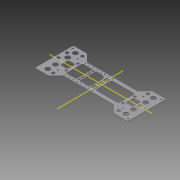
# Autodesk Inventor part: piastraX
Saved by Autodesk Inventor 2014 SP1 (Build 180222100, 222)
## iProperties
Created: 2015-04-08
Part Number: piastraX
Material: Generic
Document SubType Name: Modeling
Designer: Giorgio Nuzzo
Density: 1 g/cm^3
Appearance: Default
Author: Giorgio Nuzzo
Autodesk Inventor part; units mm, degrees
(part 1 of 6)
ref_plane "YZ Plane" through (0, 0, 0) normal (1, 0, 0) x (0, 1, 0)
ref_plane "XZ Plane" through (0, 0, 0) normal (0, 1, 0) x (-1, 0, 0)
ref_plane "XY Plane" through (0, 0, 0) normal (0, 0, 1) x (1, 0, 0)
sketch "Sketch1" plane through (0, 0, 0) normal (0, 0, 1) x (1, 0, 0)
  line L0 (224.6643, 218.6959) -> (272.1277, 218.6959)
  spline S0 degree 3 poles (272.1277, 218.6959) (273.7845, 218.6959) (275.1277, 217.3526) (275.1277, 215.6959) knots 1 1 1 1 2 2 2 2
  line L1 (272.1277, 218.6959) -> (273.7845, 218.6959) construction
  line L2 (273.7845, 218.6959) -> (275.1277, 217.3526) construction
  line L3 (275.1277, 217.3526) -> (275.1277, 215.6959) construction
  line L4 (275.1277, 215.6959) -> (275.1277, 81.696)
  spline S1 degree 3 poles (275.1277, 81.696) (275.1277, 80.0389) (273.7845, 78.696) (272.1277, 78.696) knots 3 3 3 3 4 4 4 4
  line L5 (275.1277, 81.696) -> (275.1277, 80.0389) construction
  line L6 (275.1277, 80.0389) -> (273.7845, 78.696) construction
  line L7 (273.7845, 78.696) -> (272.1277, 78.696) construction
  line L8 (272.1277, 78.696) -> (224.6664, 78.696)
  line L9 (224.6664, 78.696) -> (197.1053, 106.2571)
  line L10 (197.1053, 106.2571) -> (12.6874, 106.2571)
  line L11 (12.6874, 106.2571) -> (-14.8739, 78.696)
  line L12 (-14.8739, 78.696) -> (-61.8722, 78.696)
  spline S2 degree 3 poles (-61.8722, 78.696) (-63.5291, 78.696) (-64.8722, 80.0389) (-64.8722, 81.696) (-64.8722, 81.696) (-64.8722, 215.6959) (-64.8722, 215.6959) (-64.8722, 217.3526) (-63.5291, 218.6959) (-61.8722, 218.6959) knots 9 9 9 9 10 10 10 11 11 11 12 12 12 12
  line L13 (-61.8722, 78.696) -> (-63.5291, 78.696) construction
  line L14 (-63.5291, 78.696) -> (-64.8722, 80.0389) construction
  line L15 (-64.8722, 80.0389) -> (-64.8722, 81.696) construction
  line L16 (-64.8722, 81.696) -> (-64.8722, 81.696) construction
  line L17 (-64.8722, 81.696) -> (-64.8722, 215.6959) construction
  line L18 (-64.8722, 215.6959) -> (-64.8722, 215.6959) construction
  line L19 (-64.8722, 215.6959) -> (-64.8722, 217.3526) construction
  line L20 (-64.8722, 217.3526) -> (-63.5291, 218.6959) construction
  line L21 (-63.5291, 218.6959) -> (-61.8722, 218.6959) construction
  line L22 (-61.8722, 218.6959) -> (-14.8718, 218.6959)
  line L23 (-14.8718, 218.6959) -> (12.6282, 191.1959)
  line L24 (12.6282, 191.1959) -> (197.1645, 191.1959)
  line L25 (197.1645, 191.1959) -> (224.6643, 218.6959)
  line L26 (-42.132, 147.4797) -> (-42.132, 158.9796)
  line L27 (-42.132, 158.9796) -> (-37.8194, 150.7141)
  line L28 (-37.8194, 150.7141) -> (-33.507, 158.9796)
  line L29 (-33.507, 158.9796) -> (-33.507, 147.4797)
  line L30 (-60.4222, 87.8958) -> (-60.4065, 88.2075)
  line L31 (-60.4065, 88.2075) -> (-60.3603, 88.5104)
  line L32 (-60.3603, 88.5104) -> (-60.285, 88.8028)
  line L33 (-60.285, 88.8028) -> (-60.1825, 89.0829)
  line L34 (-60.1825, 89.0829) -> (-60.054, 89.3496)
  line L35 (-60.054, 89.3496) -> (-59.9013, 89.6011)
  line L36 (-59.9013, 89.6011) -> (-59.7257, 89.836)
  line L37 (-59.7257, 89.836) -> (-59.5288, 90.0524)
  line L38 (-59.5288, 90.0524) -> (-59.3123, 90.2494)
  line L39 (-59.3123, 90.2494) -> (-59.0775, 90.4248)
  line L40 (-59.0775, 90.4248) -> (-58.826, 90.5778)
  line L41 (-58.826, 90.5778) -> (-58.5594, 90.7063)
  line L42 (-58.5594, 90.7063) -> (-58.2791, 90.8086)
  line L43 (-58.2791, 90.8086) -> (-57.987, 90.884)
  line L44 (-57.987, 90.884) -> (-57.684, 90.9302)
  line L45 (-57.684, 90.9302) -> (-57.3722, 90.9457)
  line L46 (-57.3722, 90.9457) -> (-57.0604, 90.9302)
  line L47 (-57.0604, 90.9302) -> (-56.7576, 90.884)
  line L48 (-56.7576, 90.884) -> (-56.4653, 90.8086)
  line L49 (-56.4653, 90.8086) -> (-56.185, 90.7063)
  line L50 (-56.185, 90.7063) -> (-55.9184, 90.5778)
  line L51 (-55.9184, 90.5778) -> (-55.6669, 90.4248)
  line L52 (-55.6669, 90.4248) -> (-55.4321, 90.2494)
  line L53 (-55.4321, 90.2494) -> (-55.2156, 90.0524)
  line L54 (-55.2156, 90.0524) -> (-55.0187, 89.836)
  line L55 (-55.0187, 89.836) -> (-54.8432, 89.6011)
  line L56 (-54.8432, 89.6011) -> (-54.6904, 89.3496)
  line L57 (-54.6904, 89.3496) -> (-54.5619, 89.0829)
  line L58 (-54.5619, 89.0829) -> (-54.4594, 88.8028)
  line L59 (-54.4594, 88.8028) -> (-54.3841, 88.5104)
  line L60 (-54.3841, 88.5104) -> (-54.3379, 88.2075)
  line L61 (-54.3379, 88.2075) -> (-54.3223, 87.8958)
  line L62 (-54.3223, 87.8958) -> (-54.3379, 87.584)
  line L63 (-54.3379, 87.584) -> (-54.3841, 87.2811)
  line L64 (-54.3841, 87.2811) -> (-54.4594, 86.989)
  line L65 (-54.4594, 86.989) -> (-54.5619, 86.7086)
  line L66 (-54.5619, 86.7086) -> (-54.6904, 86.4419)
  line L67 (-54.6904, 86.4419) -> (-54.8432, 86.1904)
  line L68 (-54.8432, 86.1904) -> (-55.0187, 85.9558)
  line L69 (-55.0187, 85.9558) -> (-55.2156, 85.7391)
  line L70 (-55.2156, 85.7391) -> (-55.4321, 85.5424)
  line L71 (-55.4321, 85.5424) -> (-55.6669, 85.3667)
  line L72 (-55.6669, 85.3667) -> (-55.9184, 85.2141)
  line L73 (-55.9184, 85.2141) -> (-56.185, 85.0856)
  line L74 (-56.185, 85.0856) -> (-56.4653, 84.9829)
  line L75 (-56.4653, 84.9829) -> (-56.7576, 84.9078)
  line L76 (-56.7576, 84.9078) -> (-57.0604, 84.8617)
  line L77 (-57.0604, 84.8617) -> (-57.3722, 84.8458)
  line L78 (-57.3722, 84.8458) -> (-57.684, 84.8617)
  line L79 (-57.684, 84.8617) -> (-57.987, 84.9078)
  line L80 (-57.987, 84.9078) -> (-58.2791, 84.9829)
  line L81 (-58.2791, 84.9829) -> (-58.5594, 85.0856)
  line L82 (-58.5594, 85.0856) -> (-58.826, 85.2141)
  line L83 (-58.826, 85.2141) -> (-59.0775, 85.3667)
  line L84 (-59.0775, 85.3667) -> (-59.3123, 85.5424)
  line L85 (-59.3123, 85.5424) -> (-59.5288, 85.7391)
  line L86 (-59.5288, 85.7391) -> (-59.7257, 85.9558)
  line L87 (-59.7257, 85.9558) -> (-59.9013, 86.1904)
  line L88 (-59.9013, 86.1904) -> (-60.054, 86.4419)
  line L89 (-60.054, 86.4419) -> (-60.1825, 86.7086)
  line L90 (-60.1825, 86.7086) -> (-60.285, 86.989)
  line L91 (-60.285, 86.989) -> (-60.3603, 87.2811)
  line L92 (-60.3603, 87.2811) -> (-60.4065, 87.584)
  line L93 (-60.4065, 87.584) -> (-60.4222, 87.8958)
  line L94 (-59.4222, 96.1919) -> (-59.4117, 96.4014)
  line L95 (-59.4117, 96.4014) -> (-59.3805, 96.605)
  line L96 (-59.3805, 96.605) -> (-59.3301, 96.8013)
  line L97 (-59.3301, 96.8013) -> (-59.2612, 96.9898)
  line L98 (-59.2612, 96.9898) -> (-59.1749, 97.1689)
  line L99 (-59.1749, 97.1689) -> (-59.0722, 97.3381)
  line L100 (-59.0722, 97.3381) -> (-58.954, 97.4959)
  line L101 (-58.954, 97.4959) -> (-58.8217, 97.6412)
  line L102 (-58.8217, 97.6412) -> (-58.6762, 97.7739)
  line L103 (-58.6762, 97.7739) -> (-58.5184, 97.8917)
  line L104 (-58.5184, 97.8917) -> (-58.3494, 97.9944)
  line L105 (-58.3494, 97.9944) -> (-58.1701, 98.0808)
  line L106 (-58.1701, 98.0808) -> (-57.9818, 98.1497)
  line L107 (-57.9818, 98.1497) -> (-57.7854, 98.2)
  line L108 (-57.7854, 98.2) -> (-57.5818, 98.2314)
  line L109 (-57.5818, 98.2314) -> (-57.3722, 98.2417)
  line L110 (-57.3722, 98.2417) -> (-57.1626, 98.2314)
  line L111 (-57.1626, 98.2314) -> (-56.9591, 98.2)
  line L112 (-56.9591, 98.2) -> (-56.7626, 98.1497)
  line L113 (-56.7626, 98.1497) -> (-56.5743, 98.0808)
  line L114 (-56.5743, 98.0808) -> (-56.395, 97.9944)
  line L115 (-56.395, 97.9944) -> (-56.226, 97.8917)
  line L116 (-56.226, 97.8917) -> (-56.0682, 97.7739)
  line L117 (-56.0682, 97.7739) -> (-55.9227, 97.6412)
  line L118 (-55.9227, 97.6412) -> (-55.7904, 97.4959)
  line L119 (-55.7904, 97.4959) -> (-55.6724, 97.3381)
  line L120 (-55.6724, 97.3381) -> (-55.5697, 97.1689)
  line L121 (-55.5697, 97.1689) -> (-55.4833, 96.9898)
  line L122 (-55.4833, 96.9898) -> (-55.4144, 96.8013)
  line L123 (-55.4144, 96.8013) -> (-55.3639, 96.605)
  line L124 (-55.3639, 96.605) -> (-55.3329, 96.4014)
  line L125 (-55.3329, 96.4014) -> (-55.3222, 96.1919)
  line L126 (-55.3222, 96.1919) -> (-55.3329, 95.9821)
  line L127 (-55.3329, 95.9821) -> (-55.3639, 95.7788)
  line L128 (-55.3639, 95.7788) -> (-55.4144, 95.5821)
  line L129 (-55.4144, 95.5821) -> (-55.4833, 95.394)
  line L130 (-55.4833, 95.394) -> (-55.5697, 95.2145)
  line L131 (-55.5697, 95.2145) -> (-55.6724, 95.0457)
  line L132 (-55.6724, 95.0457) -> (-55.7904, 94.8879)
  line L133 (-55.7904, 94.8879) -> (-55.9227, 94.7422)
  line L134 (-55.9227, 94.7422) -> (-56.0682, 94.6099)
  line L135 (-56.0682, 94.6099) -> (-56.226, 94.4921)
  line L136 (-56.226, 94.4921) -> (-56.395, 94.3894)
  line L137 (-56.395, 94.3894) -> (-56.5743, 94.3029)
  line L138 (-56.5743, 94.3029) -> (-56.7626, 94.234)
  line L139 (-56.7626, 94.234) -> (-56.9591, 94.1834)
  line L140 (-56.9591, 94.1834) -> (-57.1626, 94.1524)
  line L141 (-57.1626, 94.1524) -> (-57.3722, 94.1417)
  line L142 (-57.3722, 94.1417) -> (-57.5818, 94.1524)
  line L143 (-57.5818, 94.1524) -> (-57.7854, 94.1834)
  line L144 (-57.7854, 94.1834) -> (-57.9818, 94.234)
  line L145 (-57.9818, 94.234) -> (-58.1701, 94.3029)
  line L146 (-58.1701, 94.3029) -> (-58.3494, 94.3894)
  line L147 (-58.3494, 94.3894) -> (-58.5184, 94.4921)
  line L148 (-58.5184, 94.4921) -> (-58.6762, 94.6099)
  line L149 (-58.6762, 94.6099) -> (-58.8217, 94.7422)
  line L150 (-58.8217, 94.7422) -> (-58.954, 94.8879)
  line L151 (-58.954, 94.8879) -> (-59.0722, 95.0457)
  line L152 (-59.0722, 95.0457) -> (-59.1749, 95.2145)
  line L153 (-59.1749, 95.2145) -> (-59.2612, 95.394)
  line L154 (-59.2612, 95.394) -> (-59.3301, 95.5821)
  line L155 (-59.3301, 95.5821) -> (-59.3805, 95.7788)
  line L156 (-59.3805, 95.7788) -> (-59.4117, 95.9821)
  line L157 (-59.4117, 95.9821) -> (-59.4222, 96.1919)
  line L158 (-60.4222, 209.4949) -> (-60.4065, 209.8067)
  line L159 (-60.4065, 209.8067) -> (-60.3603, 210.1095)
  line L160 (-60.3603, 210.1095) -> (-60.285, 210.4018)
  line L161 (-60.285, 210.4018) -> (-60.1825, 210.6821)
  line L162 (-60.1825, 210.6821) -> (-60.054, 210.9487)
  line L163 (-60.054, 210.9487) -> (-59.9013, 211.2002)
  line L164 (-59.9013, 211.2002) -> (-59.7257, 211.435)
  line L165 (-59.7257, 211.435) -> (-59.5288, 211.6515)
  line L166 (-59.5288, 211.6515) -> (-59.3123, 211.8484)
  line L167 (-59.3123, 211.8484) -> (-59.0775, 212.0239)
  line L168 (-59.0775, 212.0239) -> (-58.826, 212.1767)
  line L169 (-58.826, 212.1767) -> (-58.5594, 212.3052)
  line L170 (-58.5594, 212.3052) -> (-58.2791, 212.4077)
  line L171 (-58.2791, 212.4077) -> (-57.987, 212.4828)
  line L172 (-57.987, 212.4828) -> (-57.684, 212.5291)
  line L173 (-57.684, 212.5291) -> (-57.3722, 212.5448)
  line L174 (-57.3722, 212.5448) -> (-57.0604, 212.5291)
  line L175 (-57.0604, 212.5291) -> (-56.7576, 212.4828)
  line L176 (-56.7576, 212.4828) -> (-56.4653, 212.4077)
  line L177 (-56.4653, 212.4077) -> (-56.185, 212.3052)
  line L178 (-56.185, 212.3052) -> (-55.9184, 212.1767)
  line L179 (-55.9184, 212.1767) -> (-55.6669, 212.0239)
  line L180 (-55.6669, 212.0239) -> (-55.4321, 211.8484)
  line L181 (-55.4321, 211.8484) -> (-55.2156, 211.6515)
  line L182 (-55.2156, 211.6515) -> (-55.0187, 211.435)
  line L183 (-55.0187, 211.435) -> (-54.8432, 211.2002)
  line L184 (-54.8432, 211.2002) -> (-54.6904, 210.9487)
  line L185 (-54.6904, 210.9487) -> (-54.5619, 210.6821)
  line L186 (-54.5619, 210.6821) -> (-54.4594, 210.4018)
  line L187 (-54.4594, 210.4018) -> (-54.3841, 210.1095)
  line L188 (-54.3841, 210.1095) -> (-54.3379, 209.8067)
  line L189 (-54.3379, 209.8067) -> (-54.3223, 209.4949)
  line L190 (-54.3223, 209.4949) -> (-54.3379, 209.1829)
  line L191 (-54.3379, 209.1829) -> (-54.3841, 208.8801)
  line L192 (-54.3841, 208.8801) -> (-54.4594, 208.5878)
  line L193 (-54.4594, 208.5878) -> (-54.5619, 208.3077)
  line L194 (-54.5619, 208.3077) -> (-54.6904, 208.041)
  line L195 (-54.6904, 208.041) -> (-54.8432, 207.7896)
  line L196 (-54.8432, 207.7896) -> (-55.0187, 207.5548)
  line L197 (-55.0187, 207.5548) -> (-55.2156, 207.3382)
  line L198 (-55.2156, 207.3382) -> (-55.4321, 207.1414)
  line L199 (-55.4321, 207.1414) -> (-55.6669, 206.9657)
  line L200 (-55.6669, 206.9657) -> (-55.9184, 206.8129)
  line L201 (-55.9184, 206.8129) -> (-56.185, 206.6845)
  line L202 (-56.185, 206.6845) -> (-56.4653, 206.5821)
  line L203 (-56.4653, 206.5821) -> (-56.7576, 206.5068)
  line L204 (-56.7576, 206.5068) -> (-57.0604, 206.4606)
  line L205 (-57.0604, 206.4606) -> (-57.3722, 206.4448)
  line L206 (-57.3722, 206.4448) -> (-57.684, 206.4606)
  line L207 (-57.684, 206.4606) -> (-57.987, 206.5068)
  line L208 (-57.987, 206.5068) -> (-58.2791, 206.5821)
  line L209 (-58.2791, 206.5821) -> (-58.5594, 206.6845)
  line L210 (-58.5594, 206.6845) -> (-58.826, 206.8129)
  line L211 (-58.826, 206.8129) -> (-59.0775, 206.9657)
  line L212 (-59.0775, 206.9657) -> (-59.3123, 207.1414)
  line L213 (-59.3123, 207.1414) -> (-59.5288, 207.3382)
  line L214 (-59.5288, 207.3382) -> (-59.7257, 207.5548)
  line L215 (-59.7257, 207.5548) -> (-59.9013, 207.7896)
  line L216 (-59.9013, 207.7896) -> (-60.054, 208.041)
  line L217 (-60.054, 208.041) -> (-60.1825, 208.3077)
  line L218 (-60.1825, 208.3077) -> (-60.285, 208.5878)
  line L219 (-60.285, 208.5878) -> (-60.3603, 208.8801)
  line L220 (-60.3603, 208.8801) -> (-60.4065, 209.1829)
  line L221 (-60.4065, 209.1829) -> (-60.4222, 209.4949)
  line L222 (-59.4222, 201.1979) -> (-59.4117, 201.4075)
  line L223 (-59.4117, 201.4075) -> (-59.3805, 201.6109)
  line L224 (-59.3805, 201.6109) -> (-59.3301, 201.8075)
  line L225 (-59.3301, 201.8075) -> (-59.2612, 201.9958)
  line L226 (-59.2612, 201.9958) -> (-59.1749, 202.1749)
  line L227 (-59.1749, 202.1749) -> (-59.0722, 202.3441)
  line L228 (-59.0722, 202.3441) -> (-58.954, 202.5019)
  line L229 (-58.954, 202.5019) -> (-58.8217, 202.6474)
  line L230 (-58.8217, 202.6474) -> (-58.6762, 202.7797)
  line L231 (-58.6762, 202.7797) -> (-58.5184, 202.8977)
  line L232 (-58.5184, 202.8977) -> (-58.3494, 203.0004)
  line L233 (-58.3494, 203.0004) -> (-58.1701, 203.0867)
  line L234 (-58.1701, 203.0867) -> (-57.9818, 203.1557)
  line L235 (-57.9818, 203.1557) -> (-57.7854, 203.2062)
  line L236 (-57.7854, 203.2062) -> (-57.5818, 203.2372)
  line L237 (-57.5818, 203.2372) -> (-57.3722, 203.2479)
  line L238 (-57.3722, 203.2479) -> (-57.1626, 203.2372)
  line L239 (-57.1626, 203.2372) -> (-56.9591, 203.2062)
  line L240 (-56.9591, 203.2062) -> (-56.7626, 203.1557)
  line L241 (-56.7626, 203.1557) -> (-56.5743, 203.0867)
  line L242 (-56.5743, 203.0867) -> (-56.395, 203.0004)
  line L243 (-56.395, 203.0004) -> (-56.226, 202.8977)
  line L244 (-56.226, 202.8977) -> (-56.0682, 202.7797)
  line L245 (-56.0682, 202.7797) -> (-55.9227, 202.6474)
  line L246 (-55.9227, 202.6474) -> (-55.7904, 202.5019)
  line L247 (-55.7904, 202.5019) -> (-55.6724, 202.3441)
  line L248 (-55.6724, 202.3441) -> (-55.5697, 202.1749)
  line L249 (-55.5697, 202.1749) -> (-55.4833, 201.9958)
  line L250 (-55.4833, 201.9958) -> (-55.4144, 201.8075)
  line L251 (-55.4144, 201.8075) -> (-55.3639, 201.6109)
  line L252 (-55.3639, 201.6109) -> (-55.3329, 201.4075)
  line L253 (-55.3329, 201.4075) -> (-55.3222, 201.1979)
  line L254 (-55.3222, 201.1979) -> (-55.3329, 200.9882)
  line L255 (-55.3329, 200.9882) -> (-55.3639, 200.7846)
  line L256 (-55.3639, 200.7846) -> (-55.4144, 200.5883)
  line L257 (-55.4144, 200.5883) -> (-55.4833, 200.3998)
  line L258 (-55.4833, 200.3998) -> (-55.5697, 200.2207)
  line L259 (-55.5697, 200.2207) -> (-55.6724, 200.0517)
  line L260 (-55.6724, 200.0517) -> (-55.7904, 199.8939)
  line L261 (-55.7904, 199.8939) -> (-55.9227, 199.7484)
  line L262 (-55.9227, 199.7484) -> (-56.0682, 199.6159)
  line L263 (-56.0682, 199.6159) -> (-56.226, 199.4979)
  line L264 (-56.226, 199.4979) -> (-56.395, 199.3952)
  line L265 (-56.395, 199.3952) -> (-56.5743, 199.3089)
  line L266 (-56.5743, 199.3089) -> (-56.7626, 199.24)
  line L267 (-56.7626, 199.24) -> (-56.9591, 199.1896)
  line L268 (-56.9591, 199.1896) -> (-57.1626, 199.1584)
  line L269 (-57.1626, 199.1584) -> (-57.3722, 199.1479)
  line L270 (-57.3722, 199.1479) -> (-57.5818, 199.1584)
  line L271 (-57.5818, 199.1584) -> (-57.7854, 199.1896)
  line L272 (-57.7854, 199.1896) -> (-57.9818, 199.24)
  line L273 (-57.9818, 199.24) -> (-58.1701, 199.3089)
  line L274 (-58.1701, 199.3089) -> (-58.3494, 199.3952)
  line L275 (-58.3494, 199.3952) -> (-58.5184, 199.4979)
  line L276 (-58.5184, 199.4979) -> (-58.6762, 199.6159)
  line L277 (-58.6762, 199.6159) -> (-58.8217, 199.7484)
  line L278 (-58.8217, 199.7484) -> (-58.954, 199.8939)
  line L279 (-58.954, 199.8939) -> (-59.0722, 200.0517)
  line L280 (-59.0722, 200.0517) -> (-59.1749, 200.2207)
  line L281 (-59.1749, 200.2207) -> (-59.2612, 200.3998)
  line L282 (-59.2612, 200.3998) -> (-59.3301, 200.5883)
  line L283 (-59.3301, 200.5883) -> (-59.3805, 200.7846)
  line L284 (-59.3805, 200.7846) -> (-59.4117, 200.9882)
  line L285 (-59.4117, 200.9882) -> (-59.4222, 201.1979)
  line L286 (-58.9311, 141.6978) -> (-58.923, 141.8563)
  line L287 (-58.923, 141.8563) -> (-58.8996, 142.0103)
  line L288 (-58.8996, 142.0103) -> (-58.8614, 142.1588)
  line L289 (-58.8614, 142.1588) -> (-58.8092, 142.3014)
  line L290 (-58.8092, 142.3014) -> (-58.6664, 142.5646)
  line L291 (-58.6664, 142.5646) -> (-58.4771, 142.794)
  line L292 (-58.4771, 142.794) -> (-58.2476, 142.9832)
  line L293 (-58.2476, 142.9832) -> (-57.9844, 143.1261)
  line L294 (-57.9844, 143.1261) -> (-57.8419, 143.1782)
  line L295 (-57.8419, 143.1782) -> (-57.6935, 143.2164)
  line L296 (-57.6935, 143.2164) -> (-57.5395, 143.2398)
  line L297 (-57.5395, 143.2398) -> (-57.381, 143.2481)
  line L298 (-57.381, 143.2481) -> (-57.2225, 143.2398)
  line L299 (-57.2225, 143.2398) -> (-57.0687, 143.2164)
  line L300 (-57.0687, 143.2164) -> (-56.92, 143.1782)
  line L301 (-56.92, 143.1782) -> (-56.7778, 143.1261)
  line L302 (-56.7778, 143.1261) -> (-56.5144, 142.9832)
  line L303 (-56.5144, 142.9832) -> (-56.2851, 142.794)
  line L304 (-56.2851, 142.794) -> (-56.0958, 142.5646)
  line L305 (-56.0958, 142.5646) -> (-55.9528, 142.3014)
  line L306 (-55.9528, 142.3014) -> (-55.9008, 142.1588)
  line L307 (-55.9008, 142.1588) -> (-55.8626, 142.0103)
  line L308 (-55.8626, 142.0103) -> (-55.839, 141.8563)
  line L309 (-55.839, 141.8563) -> (-55.831, 141.6978)
  line L310 (-55.831, 141.6978) -> (-55.839, 141.5393)
  line L311 (-55.839, 141.5393) -> (-55.8626, 141.3857)
  line L312 (-55.8626, 141.3857) -> (-55.9008, 141.2369)
  line L313 (-55.9008, 141.2369) -> (-55.9528, 141.0946)
  line L314 (-55.9528, 141.0946) -> (-56.0958, 140.8314)
  line L315 (-56.0958, 140.8314) -> (-56.2851, 140.6019)
  line L316 (-56.2851, 140.6019) -> (-56.5144, 140.4128)
  line L317 (-56.5144, 140.4128) -> (-56.7778, 140.2698)
  line L318 (-56.7778, 140.2698) -> (-56.92, 140.2175)
  line L319 (-56.92, 140.2175) -> (-57.0687, 140.1796)
  line L320 (-57.0687, 140.1796) -> (-57.2225, 140.1558)
  line L321 (-57.2225, 140.1558) -> (-57.381, 140.1479)
  line L322 (-57.381, 140.1479) -> (-57.5395, 140.1558)
  line L323 (-57.5395, 140.1558) -> (-57.6935, 140.1796)
  line L324 (-57.6935, 140.1796) -> (-57.8419, 140.2175)
  line L325 (-57.8419, 140.2175) -> (-57.9844, 140.2698)
  line L326 (-57.9844, 140.2698) -> (-58.2476, 140.4128)
  line L327 (-58.2476, 140.4128) -> (-58.4771, 140.6019)
  line L328 (-58.4771, 140.6019) -> (-58.6664, 140.8314)
  line L329 (-58.6664, 140.8314) -> (-58.8092, 141.0946)
  line L330 (-58.8092, 141.0946) -> (-58.8614, 141.2369)
  line L331 (-58.8614, 141.2369) -> (-58.8996, 141.3857)
  line L332 (-58.8996, 141.3857) -> (-58.923, 141.5393)
  line L333 (-58.923, 141.5393) -> (-58.9311, 141.6978)
  line L334 (-40.4241, 141.6978) -> (-40.4161, 141.8563)
  line L335 (-40.4161, 141.8563) -> (-40.3925, 142.0103)
  line L336 (-40.3925, 142.0103) -> (-40.3545, 142.1588)
  line L337 (-40.3545, 142.1588) -> (-40.3023, 142.3014)
  line L338 (-40.3023, 142.3014) -> (-40.1593, 142.5646)
  line L339 (-40.1593, 142.5646) -> (-39.9702, 142.794)
  line L340 (-39.9702, 142.794) -> (-39.7407, 142.9832)
  line L341 (-39.7407, 142.9832) -> (-39.4773, 143.1261)
  line L342 (-39.4773, 143.1261) -> (-39.3351, 143.1782)
  line L343 (-39.3351, 143.1782) -> (-39.1864, 143.2164)
  line L344 (-39.1864, 143.2164) -> (-39.0326, 143.2398)
  line L345 (-39.0326, 143.2398) -> (-38.8741, 143.2481)
  line L346 (-38.8741, 143.2481) -> (-38.7156, 143.2398)
  line L347 (-38.7156, 143.2398) -> (-38.5616, 143.2164)
  line L348 (-38.5616, 143.2164) -> (-38.4132, 143.1782)
  line L349 (-38.4132, 143.1782) -> (-38.2707, 143.1261)
  line L350 (-38.2707, 143.1261) -> (-38.0075, 142.9832)
  line L351 (-38.0075, 142.9832) -> (-37.7781, 142.794)
  line L352 (-37.7781, 142.794) -> (-37.5887, 142.5646)
  line L353 (-37.5887, 142.5646) -> (-37.4459, 142.3014)
  line L354 (-37.4459, 142.3014) -> (-37.3938, 142.1588)
  line L355 (-37.3938, 142.1588) -> (-37.3555, 142.0103)
  line L356 (-37.3555, 142.0103) -> (-37.3321, 141.8563)
  line L357 (-37.3321, 141.8563) -> (-37.324, 141.6978)
  line L358 (-37.324, 141.6978) -> (-37.3321, 141.5393)
  line L359 (-37.3321, 141.5393) -> (-37.3555, 141.3857)
  line L360 (-37.3555, 141.3857) -> (-37.3938, 141.2369)
  line L361 (-37.3938, 141.2369) -> (-37.4459, 141.0946)
  line L362 (-37.4459, 141.0946) -> (-37.5887, 140.8314)
  line L363 (-37.5887, 140.8314) -> (-37.7781, 140.6019)
  line L364 (-37.7781, 140.6019) -> (-38.0075, 140.4128)
  line L365 (-38.0075, 140.4128) -> (-38.2707, 140.2698)
  line L366 (-38.2707, 140.2698) -> (-38.4132, 140.2175)
  line L367 (-38.4132, 140.2175) -> (-38.5616, 140.1796)
  line L368 (-38.5616, 140.1796) -> (-38.7156, 140.1558)
  line L369 (-38.7156, 140.1558) -> (-38.8741, 140.1479)
  line L370 (-38.8741, 140.1479) -> (-39.0326, 140.1558)
  line L371 (-39.0326, 140.1558) -> (-39.1864, 140.1796)
  line L372 (-39.1864, 140.1796) -> (-39.3351, 140.2175)
  line L373 (-39.3351, 140.2175) -> (-39.4773, 140.2698)
  line L374 (-39.4773, 140.2698) -> (-39.7407, 140.4128)
  line L375 (-39.7407, 140.4128) -> (-39.9702, 140.6019)
  line L376 (-39.9702, 140.6019) -> (-40.1593, 140.8314)
  line L377 (-40.1593, 140.8314) -> (-40.3023, 141.0946)
  line L378 (-40.3023, 141.0946) -> (-40.3545, 141.2369)
  line L379 (-40.3545, 141.2369) -> (-40.3925, 141.3857)
  line L380 (-40.3925, 141.3857) -> (-40.4161, 141.5393)
  line L381 (-40.4161, 141.5393) -> (-40.4241, 141.6978)
  line L382 (-55.4743, 115.728) -> (-55.466, 115.8913)
  line L383 (-55.466, 115.8913) -> (-55.4417, 116.0505)
  line L384 (-55.4417, 116.0505) -> (-55.4023, 116.2038)
  line L385 (-55.4023, 116.2038) -> (-55.3486, 116.3505)
  line L386 (-55.3486, 116.3505) -> (-55.281, 116.4904)
  line L387 (-55.281, 116.4904) -> (-55.2009, 116.6223)
  line L388 (-55.2009, 116.6223) -> (-55.0056, 116.8594)
  line L389 (-55.0056, 116.8594) -> (-54.7687, 117.0547)
  line L390 (-54.7687, 117.0547) -> (-54.6368, 117.1346)
  line L391 (-54.6368, 117.1346) -> (-54.4969, 117.2021)
  line L392 (-54.4969, 117.2021) -> (-54.35, 117.2559)
  line L393 (-54.35, 117.2559) -> (-54.1967, 117.2952)
  line L394 (-54.1967, 117.2952) -> (-54.0379, 117.3196)
  line L395 (-54.0379, 117.3196) -> (-53.8742, 117.3279)
  line L396 (-53.8742, 117.3279) -> (-53.7106, 117.3196)
  line L397 (-53.7106, 117.3196) -> (-53.5518, 117.2952)
  line L398 (-53.5518, 117.2952) -> (-53.3985, 117.2559)
  line L399 (-53.3985, 117.2559) -> (-53.2514, 117.2021)
  line L400 (-53.2514, 117.2021) -> (-53.1115, 117.1346)
  line L401 (-53.1115, 117.1346) -> (-52.9797, 117.0547)
  line L402 (-52.9797, 117.0547) -> (-52.7429, 116.8594)
  line L403 (-52.7429, 116.8594) -> (-52.5475, 116.6223)
  line L404 (-52.5475, 116.6223) -> (-52.4673, 116.4904)
  line L405 (-52.4673, 116.4904) -> (-52.3999, 116.3505)
  line L406 (-52.3999, 116.3505) -> (-52.3462, 116.2038)
  line L407 (-52.3462, 116.2038) -> (-52.3067, 116.0505)
  line L408 (-52.3067, 116.0505) -> (-52.2824, 115.8913)
  line L409 (-52.2824, 115.8913) -> (-52.2742, 115.728)
  line L410 (-52.2742, 115.728) -> (-52.2824, 115.5644)
  line L411 (-52.2824, 115.5644) -> (-52.3067, 115.4055)
  line L412 (-52.3067, 115.4055) -> (-52.3462, 115.2519)
  line L413 (-52.3462, 115.2519) -> (-52.3999, 115.1051)
  line L414 (-52.3999, 115.1051) -> (-52.4673, 114.9652)
  line L415 (-52.4673, 114.9652) -> (-52.5475, 114.8333)
  line L416 (-52.5475, 114.8333) -> (-52.7429, 114.5966)
  line L417 (-52.7429, 114.5966) -> (-52.9797, 114.4009)
  line L418 (-52.9797, 114.4009) -> (-53.1115, 114.321)
  line L419 (-53.1115, 114.321) -> (-53.2514, 114.2535)
  line L420 (-53.2514, 114.2535) -> (-53.3985, 114.1997)
  line L421 (-53.3985, 114.1997) -> (-53.5518, 114.1605)
  line L422 (-53.5518, 114.1605) -> (-53.7106, 114.136)
  line L423 (-53.7106, 114.136) -> (-53.8742, 114.1277)
  line L424 (-53.8742, 114.1277) -> (-54.0379, 114.136)
  line L425 (-54.0379, 114.136) -> (-54.1967, 114.1605)
  line L426 (-54.1967, 114.1605) -> (-54.35, 114.1997)
  line L427 (-54.35, 114.1997) -> (-54.4969, 114.2535)
  line L428 (-54.4969, 114.2535) -> (-54.6368, 114.321)
  line L429 (-54.6368, 114.321) -> (-54.7687, 114.4009)
  line L430 (-54.7687, 114.4009) -> (-55.0056, 114.5966)
  line L431 (-55.0056, 114.5966) -> (-55.2009, 114.8333)
  line L432 (-55.2009, 114.8333) -> (-55.281, 114.9652)
  line L433 (-55.281, 114.9652) -> (-55.3486, 115.1051)
  line L434 (-55.3486, 115.1051) -> (-55.4023, 115.2519)
  line L435 (-55.4023, 115.2519) -> (-55.4417, 115.4055)
  line L436 (-55.4417, 115.4055) -> (-55.466, 115.5644)
  line L437 (-55.466, 115.5644) -> (-55.4743, 115.728)
  line L438 (-59.8744, 185.1995) -> (-59.8665, 185.5082)
  line L439 (-59.8665, 185.5082) -> (-59.8434, 185.8129)
  line L440 (-59.8434, 185.8129) -> (-59.8051, 186.1132)
  line L441 (-59.8051, 186.1132) -> (-59.7524, 186.4086)
  line L442 (-59.7524, 186.4086) -> (-59.6046, 186.9838)
  line L443 (-59.6046, 186.9838) -> (-59.4027, 187.535)
  line L444 (-59.4027, 187.535) -> (-59.1502, 188.0595)
  line L445 (-59.1502, 188.0595) -> (-58.8496, 188.5542)
  line L446 (-58.8496, 188.5542) -> (-58.5043, 189.016)
  line L447 (-58.5043, 189.016) -> (-58.117, 189.4422)
  line L448 (-58.117, 189.4422) -> (-57.6909, 189.8294)
  line L449 (-57.6909, 189.8294) -> (-57.2289, 190.1748)
  line L450 (-57.2289, 190.1748) -> (-56.7343, 190.4754)
  line L451 (-56.7343, 190.4754) -> (-56.2098, 190.7281)
  line L452 (-56.2098, 190.7281) -> (-55.6586, 190.9298)
  line L453 (-55.6586, 190.9298) -> (-55.0835, 191.0776)
  line L454 (-55.0835, 191.0776) -> (-54.788, 191.1303)
  line L455 (-54.788, 191.1303) -> (-54.4878, 191.1685)
  line L456 (-54.4878, 191.1685) -> (-54.1831, 191.1916)
  line L457 (-54.1831, 191.1916) -> (-53.8744, 191.1995)
  line L458 (-53.8744, 191.1995) -> (-53.5656, 191.1916)
  line L459 (-53.5656, 191.1916) -> (-53.2608, 191.1685)
  line L460 (-53.2608, 191.1685) -> (-52.9606, 191.1303)
  line L461 (-52.9606, 191.1303) -> (-52.6652, 191.0776)
  line L462 (-52.6652, 191.0776) -> (-52.0902, 190.9298)
  line L463 (-52.0902, 190.9298) -> (-51.5388, 190.7281)
  line L464 (-51.5388, 190.7281) -> (-51.0143, 190.4754)
  line L465 (-51.0143, 190.4754) -> (-50.5197, 190.1748)
  line L466 (-50.5197, 190.1748) -> (-50.0578, 189.8294)
  line L467 (-50.0578, 189.8294) -> (-49.6316, 189.4422)
  line L468 (-49.6316, 189.4422) -> (-49.2444, 189.016)
  line L469 (-49.2444, 189.016) -> (-48.899, 188.5542)
  line L470 (-48.899, 188.5542) -> (-48.5984, 188.0595)
  line L471 (-48.5984, 188.0595) -> (-48.3459, 187.535)
  line L472 (-48.3459, 187.535) -> (-48.144, 186.9838)
  line L473 (-48.144, 186.9838) -> (-47.9962, 186.4086)
  line L474 (-47.9962, 186.4086) -> (-47.9435, 186.1132)
  line L475 (-47.9435, 186.1132) -> (-47.9053, 185.8129)
  line L476 (-47.9053, 185.8129) -> (-47.8822, 185.5082)
  line L477 (-47.8822, 185.5082) -> (-47.8743, 185.1995)
  line L478 (-47.8743, 185.1995) -> (-47.8822, 184.8907)
  line L479 (-47.8822, 184.8907) -> (-47.9053, 184.586)
  line L480 (-47.9053, 184.586) -> (-47.9435, 184.2857)
  line L481 (-47.9435, 184.2857) -> (-47.9962, 183.9903)
  line L482 (-47.9962, 183.9903) -> (-48.144, 183.4153)
  line L483 (-48.144, 183.4153) -> (-48.3459, 182.8639)
  line L484 (-48.3459, 182.8639) -> (-48.5984, 182.3396)
  line L485 (-48.5984, 182.3396) -> (-48.899, 181.8449)
  line L486 (-48.899, 181.8449) -> (-49.2444, 181.3829)
  line L487 (-49.2444, 181.3829) -> (-49.6316, 180.9569)
  line L488 (-49.6316, 180.9569) -> (-50.0578, 180.5695)
  line L489 (-50.0578, 180.5695) -> (-50.5197, 180.2241)
  line L490 (-50.5197, 180.2241) -> (-51.0143, 179.9236)
  line L491 (-51.0143, 179.9236) -> (-51.5388, 179.671)
  line L492 (-51.5388, 179.671) -> (-52.0902, 179.4691)
  line L493 (-52.0902, 179.4691) -> (-52.6652, 179.3214)
  line L494 (-52.6652, 179.3214) -> (-52.9606, 179.2686)
  line L495 (-52.9606, 179.2686) -> (-53.2608, 179.2304)
  line L496 (-53.2608, 179.2304) -> (-53.5656, 179.2073)
  line L497 (-53.5656, 179.2073) -> (-53.8744, 179.1994)
  line L498 (-53.8744, 179.1994) -> (-54.1831, 179.2073)
  line L499 (-54.1831, 179.2073) -> (-54.4878, 179.2304)
  line L500 (-54.4878, 179.2304) -> (-54.788, 179.2686)
  line L501 (-54.788, 179.2686) -> (-55.0835, 179.3214)
  line L502 (-55.0835, 179.3214) -> (-55.6586, 179.4691)
  line L503 (-55.6586, 179.4691) -> (-56.2098, 179.671)
  line L504 (-56.2098, 179.671) -> (-56.7343, 179.9236)
  line L505 (-56.7343, 179.9236) -> (-57.2289, 180.2241)
  line L506 (-57.2289, 180.2241) -> (-57.6909, 180.5695)
  line L507 (-57.6909, 180.5695) -> (-58.117, 180.9569)
  line L508 (-58.117, 180.9569) -> (-58.5043, 181.3829)
  line L509 (-58.5043, 181.3829) -> (-58.8496, 181.8449)
  line L510 (-58.8496, 181.8449) -> (-59.1502, 182.3396)
  line L511 (-59.1502, 182.3396) -> (-59.4027, 182.8639)
  line L512 (-59.4027, 182.8639) -> (-59.6046, 183.4153)
  line L513 (-59.6046, 183.4153) -> (-59.7524, 183.9903)
  line L514 (-59.7524, 183.9903) -> (-59.8051, 184.2857)
  line L515 (-59.8051, 184.2857) -> (-59.8434, 184.586)
  line L516 (-59.8434, 184.586) -> (-59.8665, 184.8907)
  line L517 (-59.8665, 184.8907) -> (-59.8744, 185.1995)
  line L518 (-59.8744, 153.3994) -> (-59.8665, 153.7081)
  line L519 (-59.8665, 153.7081) -> (-59.8434, 154.0128)
  line L520 (-59.8434, 154.0128) -> (-59.8051, 154.3131)
  line L521 (-59.8051, 154.3131) -> (-59.7524, 154.6087)
  line L522 (-59.7524, 154.6087) -> (-59.6046, 155.1836)
  line L523 (-59.6046, 155.1836) -> (-59.4027, 155.7349)
  line L524 (-59.4027, 155.7349) -> (-59.1502, 156.2594)
  line L525 (-59.1502, 156.2594) -> (-58.8496, 156.7541)
  line L526 (-58.8496, 156.7541) -> (-58.5043, 157.2159)
  line L527 (-58.5043, 157.2159) -> (-58.117, 157.6421)
  line L528 (-58.117, 157.6421) -> (-57.6909, 158.0293)
  line L529 (-57.6909, 158.0293) -> (-57.2289, 158.3747)
  line L530 (-57.2289, 158.3747) -> (-56.7343, 158.6752)
  line L531 (-56.7343, 158.6752) -> (-56.2098, 158.9279)
  line L532 (-56.2098, 158.9279) -> (-55.6586, 159.1296)
  line L533 (-55.6586, 159.1296) -> (-55.0835, 159.2774)
  line L534 (-55.0835, 159.2774) -> (-54.788, 159.3303)
  line L535 (-54.788, 159.3303) -> (-54.4878, 159.3684)
  line L536 (-54.4878, 159.3684) -> (-54.1831, 159.3916)
  line L537 (-54.1831, 159.3916) -> (-53.8744, 159.3994)
  line L538 (-53.8744, 159.3994) -> (-53.5656, 159.3916)
  line L539 (-53.5656, 159.3916) -> (-53.2608, 159.3684)
  line L540 (-53.2608, 159.3684) -> (-52.9606, 159.3303)
  line L541 (-52.9606, 159.3303) -> (-52.6652, 159.2774)
  line L542 (-52.6652, 159.2774) -> (-52.0902, 159.1296)
  line L543 (-52.0902, 159.1296) -> (-51.5388, 158.9279)
  line L544 (-51.5388, 158.9279) -> (-51.0143, 158.6752)
  line L545 (-51.0143, 158.6752) -> (-50.5197, 158.3747)
  line L546 (-50.5197, 158.3747) -> (-50.0578, 158.0293)
  line L547 (-50.0578, 158.0293) -> (-49.6316, 157.6421)
  line L548 (-49.6316, 157.6421) -> (-49.2444, 157.2159)
  line L549 (-49.2444, 157.2159) -> (-48.899, 156.7541)
  line L550 (-48.899, 156.7541) -> (-48.5984, 156.2594)
  line L551 (-48.5984, 156.2594) -> (-48.3459, 155.7349)
  line L552 (-48.3459, 155.7349) -> (-48.144, 155.1836)
  line L553 (-48.144, 155.1836) -> (-47.9962, 154.6087)
  line L554 (-47.9962, 154.6087) -> (-47.9435, 154.3131)
  line L555 (-47.9435, 154.3131) -> (-47.9053, 154.0128)
  line L556 (-47.9053, 154.0128) -> (-47.8822, 153.7081)
  line L557 (-47.8822, 153.7081) -> (-47.8743, 153.3994)
  line L558 (-47.8743, 153.3994) -> (-47.8822, 153.0906)
  line L559 (-47.8822, 153.0906) -> (-47.9053, 152.7859)
  line L560 (-47.9053, 152.7859) -> (-47.9435, 152.4856)
  line L561 (-47.9435, 152.4856) -> (-47.9962, 152.1902)
  line L562 (-47.9962, 152.1902) -> (-48.144, 151.6152)
  line L563 (-48.144, 151.6152) -> (-48.3459, 151.064)
  line L564 (-48.3459, 151.064) -> (-48.5984, 150.5395)
  line L565 (-48.5984, 150.5395) -> (-48.899, 150.0448)
  line L566 (-48.899, 150.0448) -> (-49.2444, 149.5828)
  line L567 (-49.2444, 149.5828) -> (-49.6316, 149.1568)
  line L568 (-49.6316, 149.1568) -> (-50.0578, 148.7696)
  line L569 (-50.0578, 148.7696) -> (-50.5197, 148.424)
  line L570 (-50.5197, 148.424) -> (-51.0143, 148.1236)
  line L571 (-51.0143, 148.1236) -> (-51.5388, 147.8711)
  line L572 (-51.5388, 147.8711) -> (-52.0902, 147.6692)
  line L573 (-52.0902, 147.6692) -> (-52.6652, 147.5214)
  line L574 (-52.6652, 147.5214) -> (-52.9606, 147.4687)
  line L575 (-52.9606, 147.4687) -> (-53.2608, 147.4304)
  line L576 (-53.2608, 147.4304) -> (-53.5656, 147.4074)
  line L577 (-53.5656, 147.4074) -> (-53.8744, 147.3994)
  line L578 (-53.8744, 147.3994) -> (-54.1831, 147.4074)
  line L579 (-54.1831, 147.4074) -> (-54.4878, 147.4304)
  line L580 (-54.4878, 147.4304) -> (-54.788, 147.4687)
  line L581 (-54.788, 147.4687) -> (-55.0835, 147.5214)
  line L582 (-55.0835, 147.5214) -> (-55.6586, 147.6692)
  line L583 (-55.6586, 147.6692) -> (-56.2098, 147.8711)
  line L584 (-56.2098, 147.8711) -> (-56.7343, 148.1236)
  line L585 (-56.7343, 148.1236) -> (-57.2289, 148.424)
  line L586 (-57.2289, 148.424) -> (-57.6909, 148.7696)
  line L587 (-57.6909, 148.7696) -> (-58.117, 149.1568)
  line L588 (-58.117, 149.1568) -> (-58.5043, 149.5828)
  line L589 (-58.5043, 149.5828) -> (-58.8496, 150.0448)
  line L590 (-58.8496, 150.0448) -> (-59.1502, 150.5395)
  line L591 (-59.1502, 150.5395) -> (-59.4027, 151.064)
  line L592 (-59.4027, 151.064) -> (-59.6046, 151.6152)
  line L593 (-59.6046, 151.6152) -> (-59.7524, 152.1902)
  line L594 (-59.7524, 152.1902) -> (-59.8051, 152.4856)
  line L595 (-59.8051, 152.4856) -> (-59.8434, 152.7859)
  line L596 (-59.8434, 152.7859) -> (-59.8665, 153.0906)
  line L597 (-59.8665, 153.0906) -> (-59.8744, 153.3994)
  line L598 (-46.8232, 199.2299) -> (-46.8114, 199.6929)
  line L599 (-46.8114, 199.6929) -> (-46.7768, 200.1501)
  line L600 (-46.7768, 200.1501) -> (-46.7195, 200.6005)
  line L601 (-46.7195, 200.6005) -> (-46.6404, 201.0437)
  line L602 (-46.6404, 201.0437) -> (-46.5398, 201.479)
  line L603 (-46.5398, 201.479) -> (-46.4185, 201.9062)
  line L604 (-46.4185, 201.9062) -> (-46.2771, 202.3243)
  line L605 (-46.2771, 202.3243) -> (-46.1159, 202.733)
  line L606 (-46.1159, 202.733) -> (-45.9357, 203.1318)
  line L607 (-45.9357, 203.1318) -> (-45.7369, 203.5197)
  line L608 (-45.7369, 203.5197) -> (-45.5202, 203.8966)
  line L609 (-45.5202, 203.8966) -> (-45.2861, 204.2618)
  line L610 (-45.2861, 204.2618) -> (-45.0353, 204.6147)
  line L611 (-45.0353, 204.6147) -> (-44.768, 204.9546)
  line L612 (-44.768, 204.9546) -> (-44.4851, 205.2812)
  line L613 (-44.4851, 205.2812) -> (-44.1871, 205.5938)
  line L614 (-44.1871, 205.5938) -> (-43.8747, 205.8918)
  line L615 (-43.8747, 205.8918) -> (-43.5481, 206.1747)
  line L616 (-43.5481, 206.1747) -> (-43.208, 206.4418)
  line L617 (-43.208, 206.4418) -> (-42.8553, 206.6928)
  line L618 (-42.8553, 206.6928) -> (-42.4901, 206.9269)
  line L619 (-42.4901, 206.9269) -> (-42.1132, 207.1436)
  line L620 (-42.1132, 207.1436) -> (-41.7251, 207.3424)
  line L621 (-41.7251, 207.3424) -> (-41.3265, 207.5226)
  line L622 (-41.3265, 207.5226) -> (-40.9177, 207.6838)
  line L623 (-40.9177, 207.6838) -> (-40.4995, 207.8252)
  line L624 (-40.4995, 207.8252) -> (-40.0725, 207.9465)
  line L625 (-40.0725, 207.9465) -> (-39.637, 208.0469)
  line L626 (-39.637, 208.0469) -> (-39.1938, 208.1261)
  line L627 (-39.1938, 208.1261) -> (-38.7434, 208.1833)
  line L628 (-38.7434, 208.1833) -> (-38.2864, 208.2181)
  line L629 (-38.2864, 208.2181) -> (-37.8232, 208.2298)
  line L630 (-37.8232, 208.2298) -> (-37.3602, 208.2181)
  line L631 (-37.3602, 208.2181) -> (-36.903, 208.1833)
  line L632 (-36.903, 208.1833) -> (-36.4526, 208.1261)
  line L633 (-36.4526, 208.1261) -> (-36.0093, 208.0469)
  line L634 (-36.0093, 208.0469) -> (-35.5741, 207.9465)
  line L635 (-35.5741, 207.9465) -> (-35.1469, 207.8252)
  line L636 (-35.1469, 207.8252) -> (-34.7288, 207.6838)
  line L637 (-34.7288, 207.6838) -> (-34.32, 207.5226)
  line L638 (-34.32, 207.5226) -> (-33.9213, 207.3424)
  line L639 (-33.9213, 207.3424) -> (-33.5334, 207.1436)
  line L640 (-33.5334, 207.1436) -> (-33.1565, 206.9269)
  line L641 (-33.1565, 206.9269) -> (-32.7913, 206.6928)
  line L642 (-32.7913, 206.6928) -> (-32.4383, 206.4418)
  line L643 (-32.4383, 206.4418) -> (-32.0983, 206.1747)
  line L644 (-32.0983, 206.1747) -> (-31.7719, 205.8918)
  line L645 (-31.7719, 205.8918) -> (-31.4592, 205.5938)
  line L646 (-31.4592, 205.5938) -> (-31.1612, 205.2812)
  line L647 (-31.1612, 205.2812) -> (-30.8784, 204.9546)
  line L648 (-30.8784, 204.9546) -> (-30.6112, 204.6147)
  line L649 (-30.6112, 204.6147) -> (-30.3602, 204.2618)
  line L650 (-30.3602, 204.2618) -> (-30.1262, 203.8966)
  line L651 (-30.1262, 203.8966) -> (-29.9095, 203.5197)
  line L652 (-29.9095, 203.5197) -> (-29.7107, 203.1318)
  line L653 (-29.7107, 203.1318) -> (-29.5305, 202.733)
  line L654 (-29.5305, 202.733) -> (-29.3693, 202.3243)
  line L655 (-29.3693, 202.3243) -> (-29.2278, 201.9062)
  line L656 (-29.2278, 201.9062) -> (-29.1066, 201.479)
  line L657 (-29.1066, 201.479) -> (-29.0062, 201.0437)
  line L658 (-29.0062, 201.0437) -> (-28.9269, 200.6005)
  line L659 (-28.9269, 200.6005) -> (-28.8697, 200.1501)
  line L660 (-28.8697, 200.1501) -> (-28.8349, 199.6929)
  line L661 (-28.8349, 199.6929) -> (-28.8232, 199.2299)
  line L662 (-28.8232, 199.2299) -> (-28.8349, 198.7667)
  line L663 (-28.8349, 198.7667) -> (-28.8697, 198.3097)
  line L664 (-28.8697, 198.3097) -> (-28.9269, 197.8592)
  line L665 (-28.9269, 197.8592) -> (-29.0062, 197.416)
  line L666 (-29.0062, 197.416) -> (-29.1066, 196.9806)
  line L667 (-29.1066, 196.9806) -> (-29.2278, 196.5535)
  line L668 (-29.2278, 196.5535) -> (-29.3693, 196.1353)
  line L669 (-29.3693, 196.1353) -> (-29.5305, 195.7266)
  line L670 (-29.5305, 195.7266) -> (-29.7107, 195.328)
  line L671 (-29.7107, 195.328) -> (-29.9095, 194.9399)
  line L672 (-29.9095, 194.9399) -> (-30.1262, 194.563)
  line L673 (-30.1262, 194.563) -> (-30.3602, 194.1978)
  line L674 (-30.3602, 194.1978) -> (-30.6112, 193.845)
  line L675 (-30.6112, 193.845) -> (-30.8784, 193.505)
  line L676 (-30.8784, 193.505) -> (-31.1612, 193.1784)
  line L677 (-31.1612, 193.1784) -> (-31.4592, 192.8659)
  line L678 (-31.4592, 192.8659) -> (-31.7719, 192.5679)
  line L679 (-31.7719, 192.5679) -> (-32.0983, 192.2849)
  line L680 (-32.0983, 192.2849) -> (-32.4383, 192.0179)
  line L681 (-32.4383, 192.0179) -> (-32.7913, 191.7669)
  line L682 (-32.7913, 191.7669) -> (-33.1565, 191.5328)
  line L683 (-33.1565, 191.5328) -> (-33.5334, 191.3161)
  line L684 (-33.5334, 191.3161) -> (-33.9213, 191.1174)
  line L685 (-33.9213, 191.1174) -> (-34.32, 190.9372)
  line L686 (-34.32, 190.9372) -> (-34.7288, 190.776)
  line L687 (-34.7288, 190.776) -> (-35.1469, 190.6344)
  line L688 (-35.1469, 190.6344) -> (-35.5741, 190.5131)
  line L689 (-35.5741, 190.5131) -> (-36.0093, 190.4127)
  line L690 (-36.0093, 190.4127) -> (-36.4526, 190.3336)
  line L691 (-36.4526, 190.3336) -> (-36.903, 190.2762)
  line L692 (-36.903, 190.2762) -> (-37.3602, 190.2416)
  line L693 (-37.3602, 190.2416) -> (-37.8232, 190.2299)
  line L694 (-37.8232, 190.2299) -> (-38.2864, 190.2416)
  line L695 (-38.2864, 190.2416) -> (-38.7434, 190.2762)
  line L696 (-38.7434, 190.2762) -> (-39.1938, 190.3336)
  line L697 (-39.1938, 190.3336) -> (-39.637, 190.4127)
  line L698 (-39.637, 190.4127) -> (-40.0725, 190.5131)
  line L699 (-40.0725, 190.5131) -> (-40.4995, 190.6344)
  line L700 (-40.4995, 190.6344) -> (-40.9177, 190.776)
  line L701 (-40.9177, 190.776) -> (-41.3265, 190.9372)
  line L702 (-41.3265, 190.9372) -> (-41.7251, 191.1174)
  line L703 (-41.7251, 191.1174) -> (-42.1132, 191.3161)
  line L704 (-42.1132, 191.3161) -> (-42.4901, 191.5328)
  line L705 (-42.4901, 191.5328) -> (-42.8553, 191.7669)
  line L706 (-42.8553, 191.7669) -> (-43.208, 192.0179)
  line L707 (-43.208, 192.0179) -> (-43.5481, 192.2849)
  line L708 (-43.5481, 192.2849) -> (-43.8747, 192.5679)
  line L709 (-43.8747, 192.5679) -> (-44.1871, 192.8659)
  line L710 (-44.1871, 192.8659) -> (-44.4851, 193.1784)
  line L711 (-44.4851, 193.1784) -> (-44.768, 193.505)
  line L712 (-44.768, 193.505) -> (-45.0353, 193.845)
  line L713 (-45.0353, 193.845) -> (-45.2861, 194.1978)
  line L714 (-45.2861, 194.1978) -> (-45.5202, 194.563)
  line L715 (-45.5202, 194.563) -> (-45.7369, 194.9399)
  line L716 (-45.7369, 194.9399) -> (-45.9357, 195.328)
  line L717 (-45.9357, 195.328) -> (-46.1159, 195.7266)
  line L718 (-46.1159, 195.7266) -> (-46.2771, 196.1353)
  line L719 (-46.2771, 196.1353) -> (-46.4185, 196.5535)
  line L720 (-46.4185, 196.5535) -> (-46.5398, 196.9806)
  line L721 (-46.5398, 196.9806) -> (-46.6404, 197.416)
  line L722 (-46.6404, 197.416) -> (-46.7195, 197.8592)
  line L723 (-46.7195, 197.8592) -> (-46.7768, 198.3097)
  line L724 (-46.7768, 198.3097) -> (-46.8114, 198.7667)
  line L725 (-46.8114, 198.7667) -> (-46.8232, 199.2299)
  line L726 (-46.8242, 171.1839) -> (-46.8125, 171.6471)
  line L727 (-46.8125, 171.6471) -> (-46.7777, 172.1041)
  line L728 (-46.7777, 172.1041) -> (-46.7205, 172.5545)
  line L729 (-46.7205, 172.5545) -> (-46.6414, 172.9977)
  line L730 (-46.6414, 172.9977) -> (-46.5408, 173.433)
  line L731 (-46.5408, 173.433) -> (-46.4196, 173.8602)
  line L732 (-46.4196, 173.8602) -> (-46.2781, 174.2784)
  line L733 (-46.2781, 174.2784) -> (-46.1169, 174.687)
  line L734 (-46.1169, 174.687) -> (-45.9367, 175.0858)
  line L735 (-45.9367, 175.0858) -> (-45.7379, 175.4737)
  line L736 (-45.7379, 175.4737) -> (-45.5213, 175.8506)
  line L737 (-45.5213, 175.8506) -> (-45.2872, 176.2158)
  line L738 (-45.2872, 176.2158) -> (-45.0362, 176.5687)
  line L739 (-45.0362, 176.5687) -> (-44.769, 176.9088)
  line L740 (-44.769, 176.9088) -> (-44.4862, 177.2352)
  line L741 (-44.4862, 177.2352) -> (-44.1882, 177.5478)
  line L742 (-44.1882, 177.5478) -> (-43.8757, 177.8458)
  line L743 (-43.8757, 177.8458) -> (-43.5491, 178.1287)
  line L744 (-43.5491, 178.1287) -> (-43.2091, 178.3958)
  line L745 (-43.2091, 178.3958) -> (-42.8561, 178.6468)
  line L746 (-42.8561, 178.6468) -> (-42.4911, 178.8809)
  line L747 (-42.4911, 178.8809) -> (-42.1142, 179.0976)
  line L748 (-42.1142, 179.0976) -> (-41.7261, 179.2964)
  line L749 (-41.7261, 179.2964) -> (-41.3274, 179.4766)
  line L750 (-41.3274, 179.4766) -> (-40.9188, 179.6378)
  line L751 (-40.9188, 179.6378) -> (-40.5005, 179.7792)
  line L752 (-40.5005, 179.7792) -> (-40.0735, 179.9005)
  line L753 (-40.0735, 179.9005) -> (-39.6381, 180.0011)
  line L754 (-39.6381, 180.0011) -> (-39.1949, 180.0801)
  line L755 (-39.1949, 180.0801) -> (-38.7444, 180.1373)
  line L756 (-38.7444, 180.1373) -> (-38.2874, 180.1721)
  line L757 (-38.2874, 180.1721) -> (-37.8242, 180.1838)
  line L758 (-37.8242, 180.1838) -> (-37.361, 180.1721)
  line L759 (-37.361, 180.1721) -> (-36.904, 180.1373)
  line L760 (-36.904, 180.1373) -> (-36.4536, 180.0801)
  line L761 (-36.4536, 180.0801) -> (-36.0104, 180.0011)
  line L762 (-36.0104, 180.0011) -> (-35.5749, 179.9005)
  line L763 (-35.5749, 179.9005) -> (-35.1479, 179.7792)
  line L764 (-35.1479, 179.7792) -> (-34.7297, 179.6378)
  line L765 (-34.7297, 179.6378) -> (-34.3211, 179.4766)
  line L766 (-34.3211, 179.4766) -> (-33.9223, 179.2964)
  line L767 (-33.9223, 179.2964) -> (-33.5342, 179.0976)
  line L768 (-33.5342, 179.0976) -> (-33.1573, 178.8809)
  line L769 (-33.1573, 178.8809) -> (-32.7923, 178.6468)
  line L770 (-32.7923, 178.6468) -> (-32.4394, 178.3958)
  line L771 (-32.4394, 178.3958) -> (-32.0993, 178.1287)
  line L772 (-32.0993, 178.1287) -> (-31.7729, 177.8458)
  line L773 (-31.7729, 177.8458) -> (-31.4603, 177.5478)
  line L774 (-31.4603, 177.5478) -> (-31.1623, 177.2352)
  line L775 (-31.1623, 177.2352) -> (-30.8794, 176.9088)
  line L776 (-30.8794, 176.9088) -> (-30.6123, 176.5687)
  line L777 (-30.6123, 176.5687) -> (-30.3613, 176.2158)
  line L778 (-30.3613, 176.2158) -> (-30.1272, 175.8506)
  line L779 (-30.1272, 175.8506) -> (-29.9105, 175.4737)
  line L780 (-29.9105, 175.4737) -> (-29.7117, 175.0858)
  line L781 (-29.7117, 175.0858) -> (-29.5315, 174.687)
  line L782 (-29.5315, 174.687) -> (-29.3703, 174.2784)
  line L783 (-29.3703, 174.2784) -> (-29.2289, 173.8602)
  line L784 (-29.2289, 173.8602) -> (-29.1076, 173.433)
  line L785 (-29.1076, 173.433) -> (-29.007, 172.9977)
  line L786 (-29.007, 172.9977) -> (-28.928, 172.5545)
  line L787 (-28.928, 172.5545) -> (-28.8708, 172.1041)
  line L788 (-28.8708, 172.1041) -> (-28.836, 171.6471)
  line L789 (-28.836, 171.6471) -> (-28.8243, 171.1839)
  line L790 (-28.8243, 171.1839) -> (-28.836, 170.7207)
  line L791 (-28.836, 170.7207) -> (-28.8708, 170.2637)
  line L792 (-28.8708, 170.2637) -> (-28.928, 169.8132)
  line L793 (-28.928, 169.8132) -> (-29.007, 169.37)
  line L794 (-29.007, 169.37) -> (-29.1076, 168.9346)
  line L795 (-29.1076, 168.9346) -> (-29.2289, 168.5075)
  line L796 (-29.2289, 168.5075) -> (-29.3703, 168.0893)
  line L797 (-29.3703, 168.0893) -> (-29.5315, 167.6805)
  line L798 (-29.5315, 167.6805) -> (-29.7117, 167.282)
  line L799 (-29.7117, 167.282) -> (-29.9105, 166.8939)
  line L800 (-29.9105, 166.8939) -> (-30.1272, 166.517)
  line L801 (-30.1272, 166.517) -> (-30.3613, 166.1518)
  line L802 (-30.3613, 166.1518) -> (-30.6123, 165.799)
  line L803 (-30.6123, 165.799) -> (-30.8794, 165.459)
  line L804 (-30.8794, 165.459) -> (-31.1623, 165.1324)
  line L805 (-31.1623, 165.1324) -> (-31.4603, 164.8199)
  line L806 (-31.4603, 164.8199) -> (-31.7729, 164.5219)
  line L807 (-31.7729, 164.5219) -> (-32.0993, 164.2391)
  line L808 (-32.0993, 164.2391) -> (-32.4394, 163.9717)
  line L809 (-32.4394, 163.9717) -> (-32.7923, 163.7209)
  line L810 (-32.7923, 163.7209) -> (-33.1573, 163.4868)
  line L811 (-33.1573, 163.4868) -> (-33.5342, 163.2701)
  line L812 (-33.5342, 163.2701) -> (-33.9223, 163.0714)
  line L813 (-33.9223, 163.0714) -> (-34.3211, 162.8912)
  line L814 (-34.3211, 162.8912) -> (-34.7297, 162.7299)
  line L815 (-34.7297, 162.7299) -> (-35.1479, 162.5885)
  line L816 (-35.1479, 162.5885) -> (-35.5749, 162.4673)
  line L817 (-35.5749, 162.4673) -> (-36.0104, 162.3667)
  line L818 (-36.0104, 162.3667) -> (-36.4536, 162.2876)
  line L819 (-36.4536, 162.2876) -> (-36.904, 162.2302)
  line L820 (-36.904, 162.2302) -> (-37.361, 162.1956)
  line L821 (-37.361, 162.1956) -> (-37.8242, 162.1839)
  line L822 (-37.8242, 162.1839) -> (-38.2874, 162.1956)
  line L823 (-38.2874, 162.1956) -> (-38.7444, 162.2302)
  line L824 (-38.7444, 162.2302) -> (-39.1949, 162.2876)
  line L825 (-39.1949, 162.2876) -> (-39.6381, 162.3667)
  line L826 (-39.6381, 162.3667) -> (-40.0735, 162.4673)
  line L827 (-40.0735, 162.4673) -> (-40.5005, 162.5885)
  line L828 (-40.5005, 162.5885) -> (-40.9188, 162.7299)
  line L829 (-40.9188, 162.7299) -> (-41.3274, 162.8912)
  line L830 (-41.3274, 162.8912) -> (-41.7261, 163.0714)
  line L831 (-41.7261, 163.0714) -> (-42.1142, 163.2701)
  line L832 (-42.1142, 163.2701) -> (-42.4911, 163.4868)
  line L833 (-42.4911, 163.4868) -> (-42.8561, 163.7209)
  line L834 (-42.8561, 163.7209) -> (-43.2091, 163.9717)
  line L835 (-43.2091, 163.9717) -> (-43.5491, 164.2391)
  line L836 (-43.5491, 164.2391) -> (-43.8757, 164.5219)
  line L837 (-43.8757, 164.5219) -> (-44.1882, 164.8199)
  line L838 (-44.1882, 164.8199) -> (-44.4862, 165.1324)
  line L839 (-44.4862, 165.1324) -> (-44.769, 165.459)
  line L840 (-44.769, 165.459) -> (-45.0362, 165.799)
  line L841 (-45.0362, 165.799) -> (-45.2872, 166.1518)
  line L842 (-45.2872, 166.1518) -> (-45.5213, 166.517)
  line L843 (-45.5213, 166.517) -> (-45.7379, 166.8939)
  line L844 (-45.7379, 166.8939) -> (-45.9367, 167.282)
  line L845 (-45.9367, 167.282) -> (-46.1169, 167.6805)
  line L846 (-46.1169, 167.6805) -> (-46.2781, 168.0893)
  line L847 (-46.2781, 168.0893) -> (-46.4196, 168.5075)
  line L848 (-46.4196, 168.5075) -> (-46.5408, 168.9346)
  line L849 (-46.5408, 168.9346) -> (-46.6414, 169.37)
  line L850 (-46.6414, 169.37) -> (-46.7205, 169.8132)
  line L851 (-46.7205, 169.8132) -> (-46.7777, 170.2637)
  line L852 (-46.7777, 170.2637) -> (-46.8125, 170.7207)
  line L853 (-46.8125, 170.7207) -> (-46.8242, 171.1839)
  line L854 (-46.8242, 126.2069) -> (-46.8125, 126.67)
  line L855 (-46.8125, 126.67) -> (-46.7777, 127.1271)
  line L856 (-46.7777, 127.1271) -> (-46.7205, 127.5774)
  line L857 (-46.7205, 127.5774) -> (-46.6414, 128.0208)
  line L858 (-46.6414, 128.0208) -> (-46.5408, 128.4559)
  line L859 (-46.5408, 128.4559) -> (-46.4196, 128.8831)
  line L860 (-46.4196, 128.8831) -> (-46.2781, 129.3013)
  line L861 (-46.2781, 129.3013) -> (-46.1169, 129.7099)
  line L862 (-46.1169, 129.7099) -> (-45.9367, 130.1089)
  line L863 (-45.9367, 130.1089) -> (-45.7379, 130.4968)
  line L864 (-45.7379, 130.4968) -> (-45.5213, 130.8737)
  line L865 (-45.5213, 130.8737) -> (-45.2872, 131.2388)